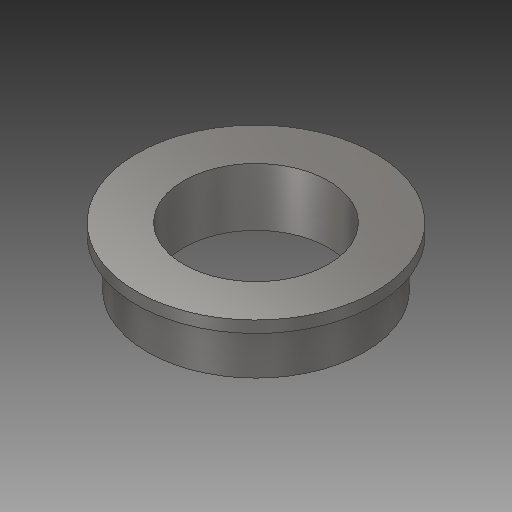
# Autodesk Inventor part: F6700ZZ Bearing
Saved by Autodesk Inventor 2019.4 (Build 234330000, 330)
## iProperties
Created: 2020-01-18
Part Number: F6700ZZ Bearing
Material: Stainless Steel
Document SubType Name: Modeling
Designer: admin
Density: 8 g/cm^3
Appearance: Semi-Polished
Author: admin
Autodesk Inventor part; units mm, degrees
ref_plane "YZ Plane" through (0, 0, 0) normal (1, 0, 0) x (0, 1, 0)
ref_plane "XZ Plane" through (0, 0, 0) normal (0, 1, 0) x (-1, 0, 0)
ref_plane "XY Plane" through (0, 0, 0) normal (0, 0, 1) x (1, 0, 0)
sketch "Sketch1" plane through (0, 0, 0) normal (0, 0, 1) x (1, 0, 0)
  line L0 (0, 0) -> (-5, 0)
  line L1 (-5, 0) -> (-5, 4)
  line L2 (-5, 4) -> (-8.25, 4)
  line L3 (-8.25, 4) -> (-8.25, 3.2)
  line L4 (-8.25, 3.2) -> (-7.5, 3.2)
  line L5 (-7.5, 3.2) -> (-7.5, 0)
  line L6 (-7.5, 0) -> (-5, 0)
  line L7 (0, -0.8) -> (0, 4.8) projected
  dimension "d0" = 4
  dimension "d1" = 5
  dimension "d2" = 7.5
  dimension "d4" = 0.8
  dimension "d6" = 8.25
  constraints: 14 end point, 6 perpendicular, 1 horizontal, 1 point on line
  measures "d0" distance of L0.end L1.end
  measures "d1" distance of L0.start L0.end
  measures "d2" distance from line of L0.start L5
  measures "d4" distance of L2.end L3.end
  measures "d6" distance between parallel lines of L7 L3
revolve "Revolution1" add sketch "Sketch1" angle 360 about axis through (0, -10, 0) along (0, 1, 0)
body "Solid1"
